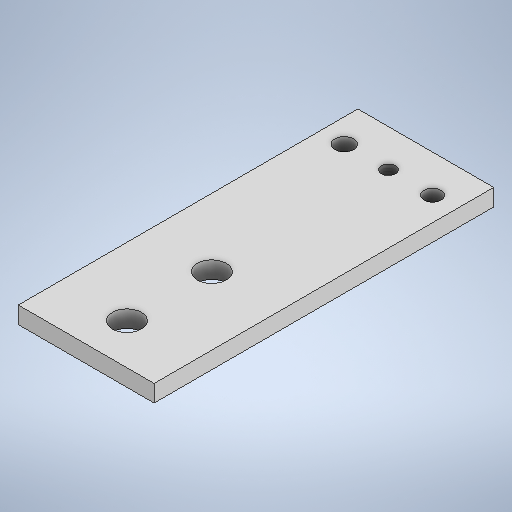
# Autodesk Inventor part: ER_Verbindungsplatte_Verschraubeinheit
Saved by Autodesk Inventor 2025.1 (Build 291241000, 241)
## iProperties
Created: 2025-06-21
Part Number: ER_Verbindungsplatte_Verschraubeinheit
Material: Generic
Document SubType Name: Modeling
Designer: Erik
Density: 1 g/cm^3
Appearance: Default
Author: Erik
Autodesk Inventor part; units mm, degrees
ref_plane "YZ Plane" through (0, 0, 0) normal (1, 0, 0) x (0, 1, 0)
ref_plane "XZ Plane" through (0, 0, 0) normal (0, 1, 0) x (-1, 0, 0)
ref_plane "XY Plane" through (0, 0, 0) normal (0, 0, 1) x (1, 0, 0)
sketch "Sketch1" plane through (0, 0, 0) normal (0, 1, 0) x (-1, 0, 0)
  line L0 (0, 0) -> (40, 0)
  line L1 (40, 0) -> (40, -100)
  line L2 (40, -100) -> (0, -100)
  line L3 (0, -100) -> (0, 0)
  dimension "d0" = 100
  dimension "d1" = 40
  constraints: 8 end point, 2 parallel, 1 horizontal, 1 perpendicular
  measures "d0" distance of L0.end L1.end
  measures "d1" distance of L1.end L2.end
extrude "Extrusion1" add sketch "Sketch1" along normal blind 5
sketch "Sketch2" plane through (0, 5, 0) normal (0, 1, 0) x (1, 0, 0)
  line L0 (-40, 100) -> (-40, 0) projected
  line L1 (-40, 89) -> (0, 89) construction
  line L2 (0, 0) -> (0, 100) projected
  line L3 (0, 100) -> (-40, 100) projected
  point P0 (-33, 89)
  point P1 (-20, 89)
  point P2 (-7, 89)
  dimension "d4" = 7
  dimension "d5" = 7
  dimension "d6" = 13
  dimension "d7" = 13
  dimension "d8" = 11
  constraints: 4 point on line, 2 end point, 1 horizontal, 1 midpoint
  measures "d4" distance from line of L0 point (-33, 89)
  measures "d5" distance from line of L2 point (-7, 89)
  measures "d6" distance of point (-7, 89) point (-20, 89)
  measures "d7" distance of point (-33, 89) point (-20, 89)
  measures "d8" distance from line of L3 point (-33, 89)
hole "Hole1" at (-33, 5, -89) direction (0, -1, 0) diameter 5.5 end through all
hole "Hole2" at (-20, 5, -89) direction (0, -1, 0) diameter 4.134 end through all thread size "M5x0.8" class "6H" standard "ISO Metric profile"
sketch "Sketch3" plane through (0, 5, 0) normal (0, 1, 0) x (1, 0, 0)
  line L0 (0, 0) -> (0, 100) projected
  line L1 (-40, 0) -> (0, 0) projected
  point P0 (-20, 12)
  point P1 (-20, 37)
  dimension "d23" = 20
  dimension "d24" = 20
  dimension "d25" = 25
  dimension "d26" = 12
  measures "d23" distance from line of L0 point (-20, 12)
  measures "d24" distance from line of L0 point (-20, 37)
  measures "d25" distance of point (-20, 37) point (-20, 12)
  measures "d26" distance from line of L1 point (-20, 12)
hole "Hole3" at (-20, 5, -12) at (-20, 5, -37) direction (0, -1, 0) diameter 8.5 end through all
hole "Hole4" at (-7, 5, -89) direction (0, -1, 0) diameter 5 end through all
equation "\"d4\" = d5"
equation "\"d6\" = d7"
equation "\"d24\" = d23"
body "Solid1"
